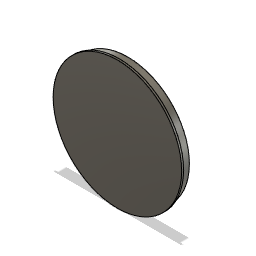
Big_Gear_ (Autodesk Fusion 360 design; units mm, degrees)
description: Spur Gear; Module: 3.0; Num Teeth: 45; Pressure Angle: 20.0; Backlash: 0.00 mm
Autodesk Fusion 360 part; units mm, degrees
(part 1 of 12)
sketch "Sketch1" plane through (0, 0, 0) normal (0, 0, 1) x (1, 0, 0) in component "Spur Gear (45 teeth)"
  circle A0 centre (0, 0) radius 63.8492
  circle A1 centre (0, 0) radius 25
extrude "Extrude1" add sketch "Sketch1" along normal blind 13 makes body 1 in component "Spur Gear (45 teeth)"
sketch "Sketch2" plane through (0, 0, 0) normal (0, 0, 1) x (1, 0, 0) in component "Spur Gear (45 teeth)"
  spline S0 degree 5 poles (63.3506, -3.1582) (63.3712, -3.1583) (63.4125, -3.1583) (63.4745, -3.1579) (63.5571, -3.1563) (63.6604, -3.1526) (63.7637, -3.1473) (63.867, -3.1403) (63.9704, -3.1319) (64.0737, -3.1219) (64.177, -3.1108) (64.2803, -3.0985) (64.3836, -3.0852) (64.4868, -3.071) (64.5901, -3.056) (64.6933, -3.0402) (64.7964, -3.0235) (64.8996, -3.0061) (65.0027, -2.9878) (65.1058, -2.9688) (65.2088, -2.949) (65.3118, -2.9284) (65.4148, -2.9072) (65.5177, -2.8853) (65.6206, -2.8627) (65.7234, -2.8395) (65.8262, -2.8156) (65.9289, -2.7911) (66.0316, -2.766) (66.1343, -2.7402) (66.2369, -2.7139) (66.3394, -2.687) (66.4419, -2.6594) (66.5443, -2.6314) (66.6467, -2.6027) (66.7491, -2.5735) (66.8514, -2.5438) (66.9536, -2.5135) (67.0558, -2.4827) (67.1579, -2.4514) (67.2599, -2.4195) (67.3619, -2.3871) (67.4639, -2.3542) (67.5657, -2.3208) (67.6675, -2.287) (67.7693, -2.2526) (67.871, -2.2177) (67.9726, -2.1824) (68.0742, -2.1465) (68.1757, -2.1102) (68.2771, -2.0735) (68.3785, -2.0362) (68.4798, -1.9985) (68.581, -1.9604) (68.6822, -1.9218) (68.7833, -1.8827) (68.8843, -1.8432) (68.9852, -1.8033) (69.0861, -1.7629) (69.1869, -1.7221) (69.2876, -1.6808) (69.3883, -1.6392) (69.4889, -1.5971) (69.5894, -1.5545) (69.6899, -1.5116) (69.7902, -1.4682) (69.8905, -1.4244) (69.9907, -1.3803) (70.0908, -1.3357) (70.1909, -1.2907) (70.2909, -1.2453) (70.3708, -1.2086) (70.4307, -1.1809) (70.4706, -1.1624) (70.4906, -1.1531) knots 0 0 0 0 0 0 0.01428571 0.02857143 0.04285714 0.05714286 0.07142857 0.08571429 0.1 0.11428571 0.12857143 0.14285714 0.15714286 0.17142857 0.18571429 0.2 0.21428571 0.22857143 0.24285714 0.25714286 0.27142857 0.28571429 0.3 0.31428571 0.32857143 0.34285714 0.35714286 0.37142857 0.38571429 0.4 0.41428571 0.42857143 0.44285714 0.45714286 0.47142857 0.48571429 0.5 0.51428571 0.52857143 0.54285714 0.55714286 0.57142857 0.58571429 0.6 0.61428571 0.62857143 0.64285714 0.65714286 0.67142857 0.68571429 0.7 0.71428571 0.72857143 0.74285714 0.75714286 0.77142857 0.78571429 0.8 0.81428571 0.82857143 0.84285714 0.85714286 0.87142857 0.88571429 0.9 0.91428571 0.92857143 0.94285714 0.95714286 0.97142857 0.98571429 1 1 1 1 1 1
  spline S1 degree 5 poles (63.3506, 3.1582) (63.3712, 3.1583) (63.4125, 3.1583) (63.4745, 3.1579) (63.5571, 3.1563) (63.6604, 3.1526) (63.7637, 3.1473) (63.867, 3.1403) (63.9704, 3.1319) (64.0737, 3.1219) (64.177, 3.1108) (64.2803, 3.0985) (64.3836, 3.0852) (64.4868, 3.071) (64.5901, 3.056) (64.6933, 3.0402) (64.7964, 3.0235) (64.8996, 3.0061) (65.0027, 2.9878) (65.1058, 2.9688) (65.2088, 2.949) (65.3118, 2.9284) (65.4148, 2.9072) (65.5177, 2.8853) (65.6206, 2.8627) (65.7234, 2.8395) (65.8262, 2.8156) (65.9289, 2.7911) (66.0316, 2.766) (66.1343, 2.7402) (66.2369, 2.7139) (66.3394, 2.687) (66.4419, 2.6594) (66.5443, 2.6314) (66.6467, 2.6027) (66.7491, 2.5735) (66.8514, 2.5438) (66.9536, 2.5135) (67.0558, 2.4827) (67.1579, 2.4514) (67.2599, 2.4195) (67.3619, 2.3871) (67.4639, 2.3542) (67.5657, 2.3208) (67.6675, 2.287) (67.7693, 2.2526) (67.871, 2.2177) (67.9726, 2.1824) (68.0742, 2.1465) (68.1757, 2.1102) (68.2771, 2.0735) (68.3785, 2.0362) (68.4798, 1.9985) (68.581, 1.9604) (68.6822, 1.9218) (68.7833, 1.8827) (68.8843, 1.8432) (68.9852, 1.8033) (69.0861, 1.7629) (69.1869, 1.7221) (69.2876, 1.6808) (69.3883, 1.6392) (69.4889, 1.5971) (69.5894, 1.5545) (69.6899, 1.5116) (69.7902, 1.4682) (69.8905, 1.4244) (69.9907, 1.3803) (70.0908, 1.3357) (70.1909, 1.2907) (70.2909, 1.2453) (70.3708, 1.2086) (70.4307, 1.1809) (70.4706, 1.1624) (70.4906, 1.1531) knots 0 0 0 0 0 0 0.01428571 0.02857143 0.04285714 0.05714286 0.07142857 0.08571429 0.1 0.11428571 0.12857143 0.14285714 0.15714286 0.17142857 0.18571429 0.2 0.21428571 0.22857143 0.24285714 0.25714286 0.27142857 0.28571429 0.3 0.31428571 0.32857143 0.34285714 0.35714286 0.37142857 0.38571429 0.4 0.41428571 0.42857143 0.44285714 0.45714286 0.47142857 0.48571429 0.5 0.51428571 0.52857143 0.54285714 0.55714286 0.57142857 0.58571429 0.6 0.61428571 0.62857143 0.64285714 0.65714286 0.67142857 0.68571429 0.7 0.71428571 0.72857143 0.74285714 0.75714286 0.77142857 0.78571429 0.8 0.81428571 0.82857143 0.84285714 0.85714286 0.87142857 0.88571429 0.9 0.91428571 0.92857143 0.94285714 0.95714286 0.97142857 0.98571429 1 1 1 1 1 1
  arc A0 (70.4906, -1.1531) -> (70.4906, 1.1531) centre (0, 0) ccw
  line L0 (63.3506, 3.1582) -> (63.3506, -3.1582)
  point P0 (63.8571, -3.1407)
  point P1 (64.3654, -3.0874)
  point P2 (64.8746, -3.0102)
  point P3 (65.3846, -2.9133)
  point P4 (65.8951, -2.7991)
  point P5 (66.406, -2.669)
  point P6 (66.917, -2.5243)
  point P7 (67.4282, -2.3657)
  point P8 (67.9393, -2.1939)
  point P9 (68.4503, -2.0094)
  point P10 (68.961, -1.8128)
  point P11 (69.4714, -1.6043)
  point P12 (69.9813, -1.3843)
  point P13 (63.8571, 3.1407)
  point P14 (64.3654, 3.0874)
  point P15 (64.8746, 3.0102)
  point P16 (65.3846, 2.9133)
  point P17 (65.8951, 2.7991)
  point P18 (66.406, 2.669)
  point P19 (66.917, 2.5243)
  point P20 (67.4282, 2.3657)
  point P21 (67.9393, 2.1939)
  point P22 (68.4503, 2.0094)
  point P23 (68.961, 1.8128)
  point P24 (69.4714, 1.6043)
  point P25 (69.9813, 1.3843)
extrude "Extrude2" add sketch "Sketch2" along normal blind 13 bodies 1 in component "Spur Gear (45 teeth)"
fillet "Fillet1" radius 1.5 2 edges at (63.7716, 3.1464, 6.5) (63.7716, -3.1464, 6.5) on bodies 1 in component "Spur Gear (45 teeth)"
pattern_circular "C-Pattern1" count 45 over 360 about axis through (0, 0, -0.0007) along (0, 0, 1) of "Extrude2", "Fillet1" in component "Spur Gear (45 teeth)"
sketch "Sketch3" plane through (0, 0, 0) normal (0, 0, 1) x (1, 0, 0) in component "Spur Gear (45 teeth)"
  circle A0 centre (0, 0) radius 67.5 construction
sketch "Sketch1 (2)" plane through (0, 0, 13) normal (0, 0, 1) x (1, 0, 0)
  arc A0 (63.688, -4.5336) -> (63.6992, -4.3741) centre (0, 0) ccw
  spline S0 degree 3 poles (64.9358, -2.9996) (64.7435, -3.0334) (64.5596, -3.1045) (64.2293, -3.3132) (64.0861, -3.4487) (63.8933, -3.7201) (63.8294, -3.8426) (63.7369, -4.1016) (63.7086, -4.2369) (63.6992, -4.3741) knots 0 0 0 0 0.058597 0.058597 0.117193 0.117193 0.158456 0.158456 0.199718 0.199718 0.199718 0.199718
  spline S1 degree 5 poles (64.9358, -2.9996) (64.9492, -2.9972) (64.9832, -2.9912) (65.0378, -2.9814) (65.113, -2.9674) (65.2088, -2.949) (65.3118, -2.9284) (65.4148, -2.9072) (65.5177, -2.8853) (65.6206, -2.8627) (65.7234, -2.8395) (65.8262, -2.8156) (65.9289, -2.7911) (66.0316, -2.766) (66.1343, -2.7402) (66.2369, -2.7139) (66.3394, -2.687) (66.4419, -2.6594) (66.5443, -2.6314) (66.6467, -2.6027) (66.7491, -2.5735) (66.8514, -2.5438) (66.9536, -2.5135) (67.0558, -2.4827) (67.1579, -2.4514) (67.2599, -2.4195) (67.3619, -2.3871) (67.4639, -2.3542) (67.5657, -2.3208) (67.6675, -2.287) (67.7693, -2.2526) (67.871, -2.2177) (67.9726, -2.1824) (68.0742, -2.1465) (68.1757, -2.1102) (68.2771, -2.0735) (68.3785, -2.0362) (68.4798, -1.9985) (68.581, -1.9604) (68.6822, -1.9218) (68.7833, -1.8827) (68.8843, -1.8432) (68.9852, -1.8033) (69.0861, -1.7629) (69.1869, -1.7221) (69.2876, -1.6808) (69.3883, -1.6392) (69.4889, -1.5971) (69.5894, -1.5545) (69.6899, -1.5116) (69.7902, -1.4682) (69.8905, -1.4244) (69.9907, -1.3803) (70.0908, -1.3357) (70.1909, -1.2907) (70.2909, -1.2453) (70.3708, -1.2086) (70.4307, -1.1809) (70.4706, -1.1624) (70.4906, -1.1531) knots 0.21931 0.21931 0.21931 0.21931 0.21931 0.21931 0.228571 0.242857 0.257143 0.271429 0.285714 0.3 0.314286 0.328571 0.342857 0.357143 0.371429 0.385714 0.4 0.414286 0.428571 0.442857 0.457143 0.471429 0.485714 0.5 0.514286 0.528571 0.542857 0.557143 0.571429 0.585714 0.6 0.614286 0.628571 0.642857 0.657143 0.671429 0.685714 0.7 0.714286 0.728571 0.742857 0.757143 0.771429 0.785714 0.8 0.814286 0.828571 0.842857 0.857143 0.871429 0.885714 0.9 0.914286 0.928571 0.942857 0.957143 0.971429 0.985714 1 1 1 1 1 1
  arc A1 (70.4906, -1.1531) -> (70.4906, 1.1531) centre (0, 0) ccw
  spline S2 degree 5 poles (70.4906, 1.1531) (70.4706, 1.1624) (70.4307, 1.1809) (70.3708, 1.2086) (70.2909, 1.2453) (70.1909, 1.2907) (70.0908, 1.3357) (69.9907, 1.3803) (69.8905, 1.4244) (69.7902, 1.4682) (69.6899, 1.5116) (69.5894, 1.5545) (69.4889, 1.5971) (69.3883, 1.6392) (69.2876, 1.6808) (69.1869, 1.7221) (69.0861, 1.7629) (68.9852, 1.8033) (68.8843, 1.8432) (68.7833, 1.8827) (68.6822, 1.9218) (68.581, 1.9604) (68.4798, 1.9985) (68.3785, 2.0362) (68.2771, 2.0735) (68.1757, 2.1102) (68.0742, 2.1465) (67.9726, 2.1824) (67.871, 2.2177) (67.7693, 2.2526) (67.6675, 2.287) (67.5657, 2.3208) (67.4639, 2.3542) (67.3619, 2.3871) (67.2599, 2.4195) (67.1579, 2.4514) (67.0558, 2.4827) (66.9536, 2.5135) (66.8514, 2.5438) (66.7491, 2.5735) (66.6467, 2.6027) (66.5443, 2.6314) (66.4419, 2.6594) (66.3394, 2.687) (66.2369, 2.7139) (66.1343, 2.7402) (66.0316, 2.766) (65.9289, 2.7911) (65.8262, 2.8156) (65.7234, 2.8395) (65.6206, 2.8627) (65.5177, 2.8853) (65.4148, 2.9072) (65.3118, 2.9284) (65.2088, 2.949) (65.113, 2.9674) (65.0378, 2.9814) (64.9832, 2.9912) (64.9492, 2.9972) (64.9358, 2.9996) knots -1 -1 -1 -1 -1 -1 -0.985714 -0.971429 -0.957143 -0.942857 -0.928571 -0.914286 -0.9 -0.885714 -0.871429 -0.857143 -0.842857 -0.828571 -0.814286 -0.8 -0.785714 -0.771429 -0.757143 -0.742857 -0.728571 -0.714286 -0.7 -0.685714 -0.671429 -0.657143 -0.642857 -0.628571 -0.614286 -0.6 -0.585714 -0.571429 -0.557143 -0.542857 -0.528571 -0.514286 -0.5 -0.485714 -0.471429 -0.457143 -0.442857 -0.428571 -0.414286 -0.4 -0.385714 -0.371429 -0.357143 -0.342857 -0.328571 -0.314286 -0.3 -0.285714 -0.271429 -0.257143 -0.242857 -0.228571 -0.21931 -0.21931 -0.21931 -0.21931 -0.21931 -0.21931
  spline S3 degree 3 poles (63.6992, 4.3741) (63.7126, 4.1793) (63.7639, 3.9889) (63.9366, 3.6385) (64.0564, 3.4818) (64.3059, 3.2615) (64.421, 3.1851) (64.6688, 3.0657) (64.8004, 3.0234) (64.9358, 2.9996) knots 0 0 0 0 0.058597 0.058597 0.117193 0.117193 0.158456 0.158456 0.199718 0.199718 0.199718 0.199718
  arc A2 (63.6992, 4.3741) -> (63.688, 4.5336) centre (0, 0) ccw
  spline S4 degree 3 poles (64.7214, 6.0669) (64.5356, 6.0067) (64.3633, 5.9107) (64.0653, 5.6581) (63.9424, 5.5039) (63.7892, 5.2084) (63.743, 5.0781) (63.6874, 4.8087) (63.6783, 4.6708) (63.688, 4.5336) knots 0 0 0 0 0.058597 0.058597 0.117193 0.117193 0.158456 0.158456 0.199718 0.199718 0.199718 0.199718
  spline S5 degree 5 poles (64.7214, 6.0669) (64.7343, 6.0711) (64.7671, 6.0818) (64.8198, 6.0992) (64.8923, 6.1235) (64.9846, 6.155) (65.0838, 6.1897) (65.1828, 6.2251) (65.2816, 6.2611) (65.3804, 6.2978) (65.4789, 6.3351) (65.5774, 6.373) (65.6757, 6.4116) (65.7739, 6.4508) (65.872, 6.4905) (65.9699, 6.5309) (66.0677, 6.5718) (66.1654, 6.6134) (66.263, 6.6554) (66.3604, 6.698) (66.4576, 6.7412) (66.5548, 6.7849) (66.6518, 6.8291) (66.7487, 6.8738) (66.8455, 6.9191) (66.9421, 6.9648) (67.0386, 7.0111) (67.1349, 7.0578) (67.2312, 7.1051) (67.3273, 7.1528) (67.4233, 7.201) (67.5191, 7.2497) (67.6148, 7.2988) (67.7104, 7.3485) (67.8059, 7.3985) (67.9012, 7.4491) (67.9964, 7.5) (68.0915, 7.5515) (68.1864, 7.6033) (68.2812, 7.6556) (68.3759, 7.7084) (68.4704, 7.7616) (68.5648, 7.8152) (68.6591, 7.8692) (68.7533, 7.9236) (68.8473, 7.9785) (68.9412, 8.0338) (69.0349, 8.0895) (69.1285, 8.1456) (69.222, 8.2021) (69.3154, 8.259) (69.4086, 8.3163) (69.5017, 8.374) (69.5946, 8.4321) (69.6874, 8.4906) (69.7801, 8.5495) (69.8542, 8.5969) (69.9096, 8.6326) (69.9466, 8.6565) (69.965, 8.6685) knots 0.21931 0.21931 0.21931 0.21931 0.21931 0.21931 0.228571 0.242857 0.257143 0.271429 0.285714 0.3 0.314286 0.328571 0.342857 0.357143 0.371429 0.385714 0.4 0.414286 0.428571 0.442857 0.457143 0.471429 0.485714 0.5 0.514286 0.528571 0.542857 0.557143 0.571429 0.585714 0.6 0.614286 0.628571 0.642857 0.657143 0.671429 0.685714 0.7 0.714286 0.728571 0.742857 0.757143 0.771429 0.785714 0.8 0.814286 0.828571 0.842857 0.857143 0.871429 0.885714 0.9 0.914286 0.928571 0.942857 0.957143 0.971429 0.985714 1 1 1 1 1 1
  arc A3 (69.965, 8.6685) -> (69.6441, 10.9523) centre (0, 0) ccw
  spline S6 degree 5 poles (69.6441, 10.9523) (69.623, 10.9587) (69.5809, 10.9715) (69.5177, 10.9906) (69.4335, 11.0157) (69.3282, 11.0468) (69.2228, 11.0774) (69.1175, 11.1076) (69.0121, 11.1375) (68.9067, 11.1669) (68.8013, 11.1958) (68.6958, 11.2244) (68.5904, 11.2525) (68.4849, 11.2802) (68.3794, 11.3075) (68.2739, 11.3343) (68.1684, 11.3607) (68.0629, 11.3866) (67.9574, 11.4121) (67.8518, 11.4372) (67.7463, 11.4618) (67.6407, 11.4859) (67.5352, 11.5096) (67.4296, 11.5329) (67.3241, 11.5556) (67.2185, 11.5779) (67.1129, 11.5997) (67.0074, 11.6211) (66.9018, 11.6419) (66.7963, 11.6623) (66.6907, 11.6822) (66.5852, 11.7016) (66.4797, 11.7205) (66.3741, 11.7389) (66.2686, 11.7567) (66.1631, 11.7741) (66.0576, 11.7909) (65.9522, 11.8072) (65.8467, 11.8229) (65.7413, 11.8382) (65.6359, 11.8528) (65.5305, 11.8669) (65.4252, 11.8805) (65.3198, 11.8935) (65.2145, 11.9059) (65.1093, 11.9177) (65.004, 11.9289) (64.8989, 11.9395) (64.7937, 11.9494) (64.6886, 11.9588) (64.5835, 11.9674) (64.4785, 11.9755) (64.3735, 11.9829) (64.2686, 11.9896) (64.1638, 11.9956) (64.0664, 12.0005) (63.9899, 12.0039) (63.9345, 12.006) (63.9, 12.0072) (63.8864, 12.0077) knots -1 -1 -1 -1 -1 -1 -0.985714 -0.971429 -0.957143 -0.942857 -0.928571 -0.914286 -0.9 -0.885714 -0.871429 -0.857143 -0.842857 -0.828571 -0.814286 -0.8 -0.785714 -0.771429 -0.757143 -0.742857 -0.728571 -0.714286 -0.7 -0.685714 -0.671429 -0.657143 -0.642857 -0.628571 -0.614286 -0.6 -0.585714 -0.571429 -0.557143 -0.542857 -0.528571 -0.514286 -0.5 -0.485714 -0.471429 -0.457143 -0.442857 -0.428571 -0.414286 -0.4 -0.385714 -0.371429 -0.357143 -0.342857 -0.328571 -0.314286 -0.3 -0.285714 -0.271429 -0.257143 -0.242857 -0.228571 -0.21931 -0.21931 -0.21931 -0.21931 -0.21931 -0.21931
  spline S7 degree 3 poles (62.4705, 13.1968) (62.5109, 13.0057) (62.5882, 12.8243) (62.808, 12.5013) (62.9484, 12.3629) (63.2261, 12.1794) (63.3508, 12.1198) (63.6128, 12.0361) (63.749, 12.0124) (63.8864, 12.0077) knots 0 0 0 0 0.058597 0.058597 0.117193 0.117193 0.158456 0.158456 0.199718 0.199718 0.199718 0.199718
  arc A4 (62.4705, 13.1968) -> (62.4373, 13.3532) centre (0, 0) ccw
  spline S8 degree 3 poles (63.2471, 15.0154) (63.0715, 14.9298) (62.9143, 14.8108) (62.6544, 14.5192) (62.5542, 14.3494) (62.4436, 14.0354) (62.416, 13.9) (62.3984, 13.6255) (62.4085, 13.4877) (62.4373, 13.3532) knots 0 0 0 0 0.058597 0.058597 0.117193 0.117193 0.158456 0.158456 0.199718 0.199718 0.199718 0.199718
  spline S9 degree 5 poles (63.2471, 15.0154) (63.2593, 15.0213) (63.2904, 15.0365) (63.3401, 15.061) (63.4086, 15.0951) (63.4956, 15.1392) (63.5889, 15.1874) (63.682, 15.2362) (63.7749, 15.2856) (63.8676, 15.3357) (63.96, 15.3864) (64.0523, 15.4376) (64.1443, 15.4895) (64.2361, 15.542) (64.3276, 15.595) (64.419, 15.6486) (64.5102, 15.7027) (64.6011, 15.7574) (64.6918, 15.8127) (64.7824, 15.8684) (64.8727, 15.9247) (64.9628, 15.9815) (65.0527, 16.0388) (65.1425, 16.0965) (65.232, 16.1548) (65.3213, 16.2136) (65.4104, 16.2728) (65.4993, 16.3325) (65.5881, 16.3927) (65.6766, 16.4533) (65.7649, 16.5144) (65.8531, 16.576) (65.941, 16.638) (66.0288, 16.7004) (66.1163, 16.7633) (66.2037, 16.8266) (66.2909, 16.8903) (66.3779, 16.9545) (66.4646, 17.019) (66.5512, 17.084) (66.6377, 17.1494) (66.7239, 17.2153) (66.8099, 17.2815) (66.8957, 17.3481) (66.9814, 17.4151) (67.0669, 17.4825) (67.1521, 17.5503) (67.2372, 17.6185) (67.3221, 17.6871) (67.4068, 17.7561) (67.4914, 17.8254) (67.5757, 17.8952) (67.6598, 17.9653) (67.7438, 18.0357) (67.8276, 18.1066) (67.9112, 18.1778) (67.9779, 18.235) (68.0278, 18.2781) (68.0611, 18.307) (68.0777, 18.3214) knots 0.21931 0.21931 0.21931 0.21931 0.21931 0.21931 0.228571 0.242857 0.257143 0.271429 0.285714 0.3 0.314286 0.328571 0.342857 0.357143 0.371429 0.385714 0.4 0.414286 0.428571 0.442857 0.457143 0.471429 0.485714 0.5 0.514286 0.528571 0.542857 0.557143 0.571429 0.585714 0.6 0.614286 0.628571 0.642857 0.657143 0.671429 0.685714 0.7 0.714286 0.728571 0.742857 0.757143 0.771429 0.785714 0.8 0.814286 0.828571 0.842857 0.857143 0.871429 0.885714 0.9 0.914286 0.928571 0.942857 0.957143 0.971429 0.985714 1 1 1 1 1 1
  arc A5 (68.0777, 18.3214) -> (67.442, 20.5383) centre (0, 0) ccw
  spline S10 degree 5 poles (67.442, 20.5383) (67.4203, 20.5417) (67.3768, 20.5485) (67.3116, 20.5586) (67.2247, 20.5718) (67.1161, 20.5879) (67.0075, 20.6036) (66.8989, 20.6188) (66.7904, 20.6337) (66.682, 20.6481) (66.5735, 20.6622) (66.4652, 20.6758) (66.3568, 20.6889) (66.2485, 20.7017) (66.1403, 20.714) (66.0321, 20.7259) (65.9239, 20.7373) (65.8158, 20.7483) (65.7078, 20.7589) (65.5998, 20.769) (65.4918, 20.7787) (65.3839, 20.7879) (65.2761, 20.7967) (65.1683, 20.805) (65.0606, 20.8129) (64.953, 20.8202) (64.8454, 20.8272) (64.7379, 20.8336) (64.6305, 20.8396) (64.5231, 20.8451) (64.4159, 20.8501) (64.3086, 20.8546) (64.2015, 20.8586) (64.0945, 20.8621) (63.9875, 20.8651) (63.8806, 20.8676) (63.7738, 20.8696) (63.6671, 20.8711) (63.5605, 20.872) (63.454, 20.8724) (63.3475, 20.8722) (63.2412, 20.8715) (63.135, 20.8703) (63.0289, 20.8685) (62.9229, 20.8661) (62.817, 20.8632) (62.7113, 20.8596) (62.6056, 20.8554) (62.5001, 20.8507) (62.3947, 20.8453) (62.2895, 20.8393) (62.1844, 20.8326) (62.0794, 20.8253) (61.9745, 20.8174) (61.8699, 20.8087) (61.7727, 20.8) (61.6966, 20.7927) (61.6414, 20.7871) (61.607, 20.7835) (61.5935, 20.7821) knots -1 -1 -1 -1 -1 -1 -0.985714 -0.971429 -0.957143 -0.942857 -0.928571 -0.914286 -0.9 -0.885714 -0.871429 -0.857143 -0.842857 -0.828571 -0.814286 -0.8 -0.785714 -0.771429 -0.757143 -0.742857 -0.728571 -0.714286 -0.7 -0.685714 -0.671429 -0.657143 -0.642857 -0.628571 -0.614286 -0.6 -0.585714 -0.571429 -0.557143 -0.542857 -0.528571 -0.514286 -0.5 -0.485714 -0.471429 -0.457143 -0.442857 -0.428571 -0.414286 -0.4 -0.385714 -0.371429 -0.357143 -0.342857 -0.328571 -0.314286 -0.3 -0.285714 -0.271429 -0.257143 -0.242857 -0.228571 -0.21931 -0.21931 -0.21931 -0.21931 -0.21931 -0.21931
  spline S11 degree 3 poles (60.0259, 21.7626) (60.0925, 21.5789) (60.1943, 21.4101) (60.4569, 21.1209) (60.6152, 21.0033) (60.9158, 20.8603) (61.0475, 20.8185) (61.3186, 20.7721) (61.4568, 20.7677) (61.5935, 20.7821) knots 0 0 0 0 0.058597 0.058597 0.117193 0.117193 0.158456 0.158456 0.199718 0.199718 0.199718 0.199718
  arc A6 (60.0259, 21.7626) -> (59.9712, 21.9128) centre (0, 0) ccw
  spline S12 degree 3 poles (60.5419, 23.6715) (60.3799, 23.5624) (60.2408, 23.4226) (60.024, 23.0977) (59.9483, 22.9156) (59.8825, 22.5893) (59.874, 22.4514) (59.8948, 22.1771) (59.924, 22.042) (59.9712, 21.9128) knots 0 0 0 0 0.058597 0.058597 0.117193 0.117193 0.158456 0.158456 0.199718 0.199718 0.199718 0.199718
  spline S13 degree 5 poles (60.5419, 23.6715) (60.5531, 23.6791) (60.5817, 23.6985) (60.6276, 23.7297) (60.6907, 23.773) (60.7707, 23.8288) (60.8564, 23.8894) (60.9418, 23.9507) (61.0269, 24.0126) (61.1117, 24.0751) (61.1962, 24.1381) (61.2804, 24.2017) (61.3643, 24.2659) (61.4479, 24.3306) (61.5312, 24.3959) (61.6142, 24.4617) (61.6969, 24.528) (61.7794, 24.5948) (61.8616, 24.6621) (61.9434, 24.73) (62.0251, 24.7983) (62.1064, 24.867) (62.1875, 24.9363) (62.2683, 25.006) (62.3488, 25.0761) (62.4291, 25.1468) (62.5091, 25.2178) (62.5889, 25.2893) (62.6683, 25.3613) (62.7476, 25.4336) (62.8265, 25.5064) (62.9053, 25.5796) (62.9837, 25.6533) (63.0619, 25.7273) (63.1399, 25.8018) (63.2176, 25.8766) (63.2951, 25.9518) (63.3723, 26.0275) (63.4492, 26.1035) (63.5259, 26.1799) (63.6024, 26.2567) (63.6786, 26.3339) (63.7546, 26.4114) (63.8303, 26.4894) (63.9058, 26.5677) (63.9811, 26.6463) (64.0561, 26.7253) (64.1309, 26.8047) (64.2054, 26.8844) (64.2797, 26.9645) (64.3537, 27.045) (64.4275, 27.1257) (64.5011, 27.2069) (64.5744, 27.2883) (64.6475, 27.3701) (64.7204, 27.4523) (64.7785, 27.5183) (64.822, 27.5679) (64.8509, 27.6011) (64.8654, 27.6177) knots 0.21931 0.21931 0.21931 0.21931 0.21931 0.21931 0.228571 0.242857 0.257143 0.271429 0.285714 0.3 0.314286 0.328571 0.342857 0.357143 0.371429 0.385714 0.4 0.414286 0.428571 0.442857 0.457143 0.471429 0.485714 0.5 0.514286 0.528571 0.542857 0.557143 0.571429 0.585714 0.6 0.614286 0.628571 0.642857 0.657143 0.671429 0.685714 0.7 0.714286 0.728571 0.742857 0.757143 0.771429 0.785714 0.8 0.814286 0.828571 0.842857 0.857143 0.871429 0.885714 0.9 0.914286 0.928571 0.942857 0.957143 0.971429 0.985714 1 1 1 1 1 1
  arc A7 (64.8654, 27.6177) -> (63.9273, 29.7245) centre (0, 0) ccw
  spline S14 degree 5 poles (63.9273, 29.7245) (63.9053, 29.7249) (63.8613, 29.7256) (63.7953, 29.7265) (63.7074, 29.7275) (63.5976, 29.7283) (63.4879, 29.7287) (63.3783, 29.7287) (63.2688, 29.7283) (63.1594, 29.7275) (63.05, 29.7263) (62.9408, 29.7247) (62.8317, 29.7227) (62.7227, 29.7202) (62.6138, 29.7173) (62.505, 29.7141) (62.3963, 29.7103) (62.2877, 29.7062) (62.1792, 29.7016) (62.0709, 29.6966) (61.9626, 29.6912) (61.8545, 29.6853) (61.7465, 29.679) (61.6386, 29.6722) (61.5309, 29.665) (61.4233, 29.6573) (61.3158, 29.6492) (61.2084, 29.6406) (61.1012, 29.6316) (60.9941, 29.6221) (60.8872, 29.6121) (60.7804, 29.6017) (60.6737, 29.5907) (60.5672, 29.5793) (60.4609, 29.5674) (60.3547, 29.555) (60.2487, 29.5421) (60.1428, 29.5287) (60.0371, 29.5148) (59.9316, 29.5003) (59.8262, 29.4854) (59.721, 29.4699) (59.616, 29.4539) (59.5112, 29.4373) (59.4065, 29.4202) (59.3021, 29.4026) (59.1979, 29.3843) (59.0938, 29.3655) (58.99, 29.3461) (58.8864, 29.3261) (58.783, 29.3055) (58.6798, 29.2843) (58.5769, 29.2624) (58.4742, 29.24) (58.3717, 29.2168) (58.2767, 29.1947) (58.2024, 29.1769) (58.1485, 29.1636) (58.115, 29.1553) (58.1018, 29.152) knots -1 -1 -1 -1 -1 -1 -0.985714 -0.971429 -0.957143 -0.942857 -0.928571 -0.914286 -0.9 -0.885714 -0.871429 -0.857143 -0.842857 -0.828571 -0.814286 -0.8 -0.785714 -0.771429 -0.757143 -0.742857 -0.728571 -0.714286 -0.7 -0.685714 -0.671429 -0.657143 -0.642857 -0.628571 -0.614286 -0.6 -0.585714 -0.571429 -0.557143 -0.542857 -0.528571 -0.514286 -0.5 -0.485714 -0.471429 -0.457143 -0.442857 -0.428571 -0.414286 -0.4 -0.385714 -0.371429 -0.357143 -0.342857 -0.328571 -0.314286 -0.3 -0.285714 -0.271429 -0.257143 -0.242857 -0.228571 -0.21931 -0.21931 -0.21931 -0.21931 -0.21931 -0.21931
  spline S15 degree 3 poles (56.413, 29.9048) (56.5045, 29.7322) (56.6288, 29.5791) (56.9291, 29.3293) (57.1022, 29.2349) (57.4198, 29.1351) (57.556, 29.1121) (57.831, 29.1039) (57.9684, 29.1187) (58.1018, 29.152) knots 0 0 0 0 0.058597 0.058597 0.117193 0.117193 0.158456 0.158456 0.199718 0.199718 0.199718 0.199718
  arc A8 (56.413, 29.9048) -> (56.3379, 30.046) centre (0, 0) ccw
  spline S16 degree 3 poles (56.6583, 31.867) (56.513, 31.7363) (56.3947, 31.5786) (56.2252, 31.2266) (56.1757, 31.0358) (56.1559, 30.7035) (56.1667, 30.5657) (56.2255, 30.297) (56.2732, 30.1673) (56.3379, 30.046) knots 0 0 0 0 0.058597 0.058597 0.117193 0.117193 0.158456 0.158456 0.199718 0.199718 0.199718 0.199718
  spline S17 degree 5 poles (56.6583, 31.867) (56.6683, 31.8761) (56.694, 31.8992) (56.7351, 31.9365) (56.7915, 31.9881) (56.8629, 32.0545) (56.9394, 32.1265) (57.0154, 32.1991) (57.0911, 32.2722) (57.1664, 32.3459) (57.2413, 32.4201) (57.3158, 32.4948) (57.3899, 32.57) (57.4637, 32.6457) (57.5371, 32.722) (57.6102, 32.7987) (57.6829, 32.8759) (57.7552, 32.9535) (57.8272, 33.0316) (57.8989, 33.1102) (57.9702, 33.1891) (58.0412, 33.2686) (58.1118, 33.3484) (58.1821, 33.4287) (58.2521, 33.5094) (58.3218, 33.5905) (58.3911, 33.672) (58.4601, 33.7539) (58.5288, 33.8362) (58.5972, 33.9189) (58.6653, 34.002) (58.7331, 34.0854) (58.8005, 34.1693) (58.8677, 34.2535) (58.9345, 34.338) (59.001, 34.423) (59.0673, 34.5082) (59.1332, 34.5939) (59.1988, 34.6799) (59.2642, 34.7662) (59.3292, 34.8529) (59.3939, 34.94) (59.4584, 35.0273) (59.5225, 35.115) (59.5864, 35.2031) (59.65, 35.2914) (59.7132, 35.3801) (59.7762, 35.4691) (59.8389, 35.5585) (59.9014, 35.6481) (59.9635, 35.7381) (60.0253, 35.8283) (60.0869, 35.9189) (60.1482, 36.0098) (60.2092, 36.101) (60.2699, 36.1925) (60.3183, 36.2659) (60.3544, 36.3211) (60.3785, 36.358) (60.3905, 36.3764) knots 0.21931 0.21931 0.21931 0.21931 0.21931 0.21931 0.228571 0.242857 0.257143 0.271429 0.285714 0.3 0.314286 0.328571 0.342857 0.357143 0.371429 0.385714 0.4 0.414286 0.428571 0.442857 0.457143 0.471429 0.485714 0.5 0.514286 0.528571 0.542857 0.557143 0.571429 0.585714 0.6 0.614286 0.628571 0.642857 0.657143 0.671429 0.685714 0.7 0.714286 0.728571 0.742857 0.757143 0.771429 0.785714 0.8 0.814286 0.828571 0.842857 0.857143 0.871429 0.885714 0.9 0.914286 0.928571 0.942857 0.957143 0.971429 0.985714 1 1 1 1 1 1
  arc A9 (60.3905, 36.3764) -> (59.1683, 38.3322) centre (0, 0) ccw
  spline S18 degree 5 poles (59.1683, 38.3322) (59.1465, 38.3295) (59.1028, 38.3241) (59.0374, 38.3158) (58.9502, 38.3045) (58.8413, 38.29) (58.7326, 38.2752) (58.6241, 38.2599) (58.5157, 38.2443) (58.4074, 38.2283) (58.2993, 38.2119) (58.1914, 38.1951) (58.0836, 38.1779) (57.976, 38.1603) (57.8686, 38.1423) (57.7613, 38.1239) (57.6541, 38.1051) (57.5472, 38.0859) (57.4404, 38.0662) (57.3338, 38.0462) (57.2274, 38.0258) (57.1211, 38.0049) (57.0151, 37.9836) (56.9092, 37.9619) (56.8035, 37.9398) (56.698, 37.9172) (56.5927, 37.8942) (56.4876, 37.8707) (56.3827, 37.8469) (56.2779, 37.8225) (56.1734, 37.7978) (56.0691, 37.7726) (55.965, 37.7469) (55.8612, 37.7208) (55.7575, 37.6942) (55.6541, 37.6671) (55.5509, 37.6396) (55.4479, 37.6116) (55.3452, 37.5831) (55.2427, 37.5541) (55.1404, 37.5246) (55.0384, 37.4947) (54.9366, 37.4642) (54.8351, 37.4332) (54.7339, 37.4017) (54.6329, 37.3697) (54.5322, 37.3371) (54.4318, 37.304) (54.3317, 37.2703) (54.2319, 37.2361) (54.1324, 37.2013) (54.0332, 37.1659) (53.9343, 37.13) (53.8357, 37.0934) (53.7375, 37.0563) (53.6465, 37.0211) (53.5753, 36.9931) (53.5238, 36.9725) (53.4918, 36.9596) (53.4792, 36.9545) knots -1 -1 -1 -1 -1 -1 -0.985714 -0.971429 -0.957143 -0.942857 -0.928571 -0.914286 -0.9 -0.885714 -0.871429 -0.857143 -0.842857 -0.828571 -0.814286 -0.8 -0.785714 -0.771429 -0.757143 -0.742857 -0.728571 -0.714286 -0.7 -0.685714 -0.671429 -0.657143 -0.642857 -0.628571 -0.614286 -0.6 -0.585714 -0.571429 -0.557143 -0.542857 -0.528571 -0.514286 -0.5 -0.485714 -0.471429 -0.457143 -0.442857 -0.428571 -0.414286 -0.4 -0.385714 -0.371429 -0.357143 -0.342857 -0.328571 -0.314286 -0.3 -0.285714 -0.271429 -0.257143 -0.242857 -0.228571 -0.21931 -0.21931 -0.21931 -0.21931 -0.21931 -0.21931
  spline S19 degree 3 poles (51.702, 37.4649) (51.8166, 37.3067) (51.9611, 37.1725) (52.2932, 36.9669) (52.4778, 36.8975) (52.8061, 36.8428) (52.9443, 36.839) (53.2177, 36.8692) (53.3517, 36.903) (53.4792, 36.9545) knots 0 0 0 0 0.058597 0.058597 0.117193 0.117193 0.158456 0.158456 0.199718 0.199718 0.199718 0.199718
  arc A10 (51.702, 37.4649) -> (51.6081, 37.5943) centre (0, 0) ccw
  spline S20 degree 3 poles (51.6718, 39.4422) (51.5462, 39.2926) (51.451, 39.1199) (51.3322, 38.7478) (51.3096, 38.5519) (51.3363, 38.2201) (51.3662, 38.0852) (51.4618, 37.8272) (51.5271, 37.7054) (51.6081, 37.5943) knots 0 0 0 0 0.058597 0.058597 0.117193 0.117193 0.158456 0.158456 0.199718 0.199718 0.199718 0.199718
  spline S21 degree 5 poles (51.6718, 39.4422) (51.6806, 39.4525) (51.7027, 39.479) (51.7382, 39.5217) (51.7869, 39.5807) (51.8484, 39.6564) (51.9141, 39.7383) (51.9793, 39.8208) (52.0441, 39.9037) (52.1084, 39.9871) (52.1722, 40.071) (52.2356, 40.1554) (52.2986, 40.2402) (52.3611, 40.3254) (52.4232, 40.4111) (52.4848, 40.4973) (52.5461, 40.5838) (52.6069, 40.6708) (52.6673, 40.7581) (52.7274, 40.8459) (52.787, 40.934) (52.8462, 41.0226) (52.9051, 41.1115) (52.9635, 41.2007) (53.0216, 41.2904) (53.0793, 41.3804) (53.1366, 41.4708) (53.1936, 41.5615) (53.2502, 41.6525) (53.3064, 41.744) (53.3622, 41.8357) (53.4177, 41.9278) (53.4728, 42.0202) (53.5276, 42.1129) (53.582, 42.2059) (53.6361, 42.2993) (53.6898, 42.393) (53.7432, 42.487) (53.7962, 42.5813) (53.8489, 42.6759) (53.9012, 42.7708) (53.9532, 42.866) (54.0049, 42.9615) (54.0562, 43.0572) (54.1072, 43.1533) (54.1578, 43.2496) (54.2082, 43.3463) (54.2582, 43.4432) (54.3078, 43.5404) (54.3572, 43.6378) (54.4062, 43.7356) (54.4548, 43.8336) (54.5032, 43.9318) (54.5512, 44.0304) (54.599, 44.1291) (54.6464, 44.2282) (54.684, 44.3076) (54.7121, 44.3673) (54.7308, 44.4072) (54.7401, 44.4271) knots 0.21931 0.21931 0.21931 0.21931 0.21931 0.21931 0.228571 0.242857 0.257143 0.271429 0.285714 0.3 0.314286 0.328571 0.342857 0.357143 0.371429 0.385714 0.4 0.414286 0.428571 0.442857 0.457143 0.471429 0.485714 0.5 0.514286 0.528571 0.542857 0.557143 0.571429 0.585714 0.6 0.614286 0.628571 0.642857 0.657143 0.671429 0.685714 0.7 0.714286 0.728571 0.742857 0.757143 0.771429 0.785714 0.8 0.814286 0.828571 0.842857 0.857143 0.871429 0.885714 0.9 0.914286 0.928571 0.942857 0.957143 0.971429 0.985714 1 1 1 1 1 1
  arc A11 (54.7401, 44.4271) -> (53.2577, 46.1938) centre (0, 0) ccw
  spline S22 degree 5 poles (53.2577, 46.1938) (53.2364, 46.1881) (53.194, 46.1766) (53.1303, 46.1593) (53.0455, 46.136) (52.9397, 46.1065) (52.8342, 46.0767) (52.7288, 46.0465) (52.6236, 46.0159) (52.5187, 45.985) (52.4139, 45.9537) (52.3094, 45.9221) (52.205, 45.89) (52.1009, 45.8576) (51.997, 45.8248) (51.8933, 45.7917) (51.7899, 45.7582) (51.6866, 45.7242) (51.5836, 45.6899) (51.4808, 45.6553) (51.3783, 45.6202) (51.276, 45.5848) (51.1739, 45.5489) (51.0721, 45.5127) (50.9705, 45.476) (50.8692, 45.439) (50.7681, 45.4016) (50.6673, 45.3637) (50.5667, 45.3255) (50.4664, 45.2868) (50.3663, 45.2478) (50.2665, 45.2083) (50.167, 45.1684) (50.0678, 45.128) (49.9689, 45.0873) (49.8702, 45.0461) (49.7718, 45.0045) (49.6738, 44.9624) (49.576, 44.9199) (49.4785, 44.8769) (49.3814, 44.8335) (49.2845, 44.7896) (49.188, 44.7453) (49.0918, 44.7005) (48.9959, 44.6552) (48.9004, 44.6094) (48.8052, 44.5632) (48.7104, 44.5164) (48.6159, 44.4691) (48.5219, 44.4213) (48.4282, 44.373) (48.3348, 44.3242) (48.2419, 44.2748) (48.1494, 44.2249) (48.0573, 44.1745) (47.9721, 44.127) (47.9055, 44.0893) (47.8573, 44.0618) (47.8274, 44.0446) (47.8157, 44.0378) knots -1 -1 -1 -1 -1 -1 -0.985714 -0.971429 -0.957143 -0.942857 -0.928571 -0.914286 -0.9 -0.885714 -0.871429 -0.857143 -0.842857 -0.828571 -0.814286 -0.8 -0.785714 -0.771429 -0.757143 -0.742857 -0.728571 -0.714286 -0.7 -0.685714 -0.671429 -0.657143 -0.642857 -0.628571 -0.614286 -0.6 -0.585714 -0.571429 -0.557143 -0.542857 -0.528571 -0.514286 -0.5 -0.485714 -0.471429 -0.457143 -0.442857 -0.428571 -0.414286 -0.4 -0.385714 -0.371429 -0.357143 -0.342857 -0.328571 -0.314286 -0.3 -0.285714 -0.271429 -0.257143 -0.242857 -0.228571 -0.21931 -0.21931 -0.21931 -0.21931 -0.21931 -0.21931
  spline S23 degree 3 poles (45.9848, 44.2958) (46.1203, 44.1552) (46.282, 44.0423) (46.6395, 43.8849) (46.8319, 43.8419) (47.1647, 43.8335) (47.302, 43.8489) (47.5686, 43.9168) (47.6966, 43.9689) (47.8157, 44.0378) knots 0 0 0 0 0.058597 0.058597 0.117193 0.117193 0.158456 0.158456 0.199718 0.199718 0.199718 0.199718
  arc A12 (45.9848, 44.2958) -> (45.8737, 44.4109) centre (0, 0) ccw
  spline S24 degree 3 poles (45.6797, 46.2496) (45.5761, 46.084) (45.5059, 45.8998) (45.44, 45.5147) (45.4449, 45.3176) (45.5175, 44.9928) (45.5658, 44.8633) (45.6964, 44.6212) (45.778, 44.5097) (45.8737, 44.4109) knots 0 0 0 0 0.058597 0.058597 0.117193 0.117193 0.158456 0.158456 0.199718 0.199718 0.199718 0.199718
  spline S25 degree 5 poles (45.6797, 46.2496) (45.6869, 46.2611) (45.7051, 46.2904) (45.7344, 46.3376) (45.7743, 46.4028) (45.8247, 46.4863) (45.8784, 46.5766) (45.9315, 46.6674) (45.9841, 46.7585) (46.0361, 46.8501) (46.0877, 46.942) (46.1387, 47.0344) (46.1892, 47.1271) (46.2393, 47.2203) (46.2888, 47.3138) (46.3379, 47.4076) (46.3865, 47.5019) (46.4347, 47.5964) (46.4823, 47.6914) (46.5296, 47.7866) (46.5764, 47.8822) (46.6227, 47.9781) (46.6686, 48.0743) (46.7141, 48.1709) (46.7591, 48.2677) (46.8037, 48.3649) (46.8479, 48.4624) (46.8917, 48.5601) (46.935, 48.6582) (46.978, 48.7565) (47.0205, 48.8551) (47.0626, 48.954) (47.1044, 49.0532) (47.1457, 49.1527) (47.1866, 49.2524) (47.2272, 49.3524) (47.2673, 49.4526) (47.3071, 49.5531) (47.3465, 49.6539) (47.3855, 49.7549) (47.4241, 49.8561) (47.4624, 49.9576) (47.5002, 50.0594) (47.5377, 50.1614) (47.5748, 50.2636) (47.6116, 50.3661) (47.648, 50.4688) (47.684, 50.5717) (47.7196, 50.6748) (47.7549, 50.7782) (47.7899, 50.8818) (47.8244, 50.9856) (47.8587, 51.0897) (47.8925, 51.1939) (47.926, 51.2984) (47.9592, 51.4031) (47.9854, 51.487) (48.0049, 51.55) (48.0179, 51.5921) (48.0243, 51.6131) knots 0.21931 0.21931 0.21931 0.21931 0.21931 0.21931 0.228571 0.242857 0.257143 0.271429 0.285714 0.3 0.314286 0.328571 0.342857 0.357143 0.371429 0.385714 0.4 0.414286 0.428571 0.442857 0.457143 0.471429 0.485714 0.5 0.514286 0.528571 0.542857 0.557143 0.571429 0.585714 0.6 0.614286 0.628571 0.642857 0.657143 0.671429 0.685714 0.7 0.714286 0.728571 0.742857 0.757143 0.771429 0.785714 0.8 0.814286 0.828571 0.842857 0.857143 0.871429 0.885714 0.9 0.914286 0.928571 0.942857 0.957143 0.971429 0.985714 1 1 1 1 1 1
  arc A13 (48.0243, 51.6131) -> (46.3105, 53.1563) centre (0, 0) ccw
  spline S26 degree 5 poles (46.3105, 53.1563) (46.2902, 53.1477) (46.2497, 53.1304) (46.1891, 53.1044) (46.1084, 53.0695) (46.0077, 53.0256) (45.9073, 52.9814) (45.8072, 52.9368) (45.7073, 52.8919) (45.6077, 52.8467) (45.5083, 52.8011) (45.4092, 52.7552) (45.3103, 52.709) (45.2117, 52.6624) (45.1134, 52.6155) (45.0153, 52.5682) (44.9175, 52.5206) (44.82, 52.4726) (44.7228, 52.4243) (44.6258, 52.3757) (44.5292, 52.3267) (44.4328, 52.2774) (44.3367, 52.2277) (44.2409, 52.1776) (44.1454, 52.1272) (44.0502, 52.0764) (43.9553, 52.0253) (43.8607, 51.9738) (43.7665, 51.9219) (43.6725, 51.8697) (43.5789, 51.8171) (43.4856, 51.7641) (43.3926, 51.7107) (43.2999, 51.657) (43.2076, 51.6028) (43.1157, 51.5483) (43.0241, 51.4934) (42.9328, 51.4381) (42.8419, 51.3824) (42.7513, 51.3263) (42.6612, 51.2697) (42.5714, 51.2128) (42.482, 51.1555) (42.3929, 51.0977) (42.3043, 51.0395) (42.2161, 50.9809) (42.1283, 50.9218) (42.0409, 50.8623) (41.9539, 50.8024) (41.8674, 50.742) (41.7813, 50.6811) (41.6957, 50.6197) (41.6106, 50.5579) (41.5259, 50.4956) (41.4417, 50.4328) (41.3639, 50.374) (41.3032, 50.3274) (41.2594, 50.2934) (41.2321, 50.2722) (41.2214, 50.2638) knots -1 -1 -1 -1 -1 -1 -0.985714 -0.971429 -0.957143 -0.942857 -0.928571 -0.914286 -0.9 -0.885714 -0.871429 -0.857143 -0.842857 -0.828571 -0.814286 -0.8 -0.785714 -0.771429 -0.757143 -0.742857 -0.728571 -0.714286 -0.7 -0.685714 -0.671429 -0.657143 -0.642857 -0.628571 -0.614286 -0.6 -0.585714 -0.571429 -0.557143 -0.542857 -0.528571 -0.514286 -0.5 -0.485714 -0.471429 -0.457143 -0.442857 -0.428571 -0.414286 -0.4 -0.385714 -0.371429 -0.357143 -0.342857 -0.328571 -0.314286 -0.3 -0.285714 -0.271429 -0.257143 -0.242857 -0.228571 -0.21931 -0.21931 -0.21931 -0.21931 -0.21931 -0.21931
  spline S27 degree 3 poles (39.3725, 50.2646) (39.5262, 50.1442) (39.702, 50.0549) (40.078, 49.9488) (40.2746, 49.933) (40.6052, 49.9709) (40.7391, 50.0054) (40.9936, 50.1097) (41.1131, 50.1791) (41.2214, 50.2638) knots 0 0 0 0 0.058597 0.058597 0.117193 0.117193 0.158456 0.158456 0.199718 0.199718 0.199718 0.199718
  arc A14 (39.3725, 50.2646) -> (39.2465, 50.363) centre (0, 0) ccw
  spline S28 degree 3 poles (38.7984, 52.1569) (38.7189, 51.9785) (38.675, 51.7863) (38.6633, 51.3958) (38.6957, 51.2013) (38.8128, 50.8897) (38.8786, 50.7682) (39.0416, 50.5466) (39.138, 50.4476) (39.2465, 50.363) knots 0 0 0 0 0.058597 0.058597 0.117193 0.117193 0.158456 0.158456 0.199718 0.199718 0.199718 0.199718
  spline S29 degree 5 poles (38.7984, 52.1569) (38.8039, 52.1693) (38.818, 52.2009) (38.8403, 52.2516) (38.8708, 52.3218) (38.9091, 52.4115) (38.9497, 52.5084) (38.9896, 52.6056) (39.029, 52.7032) (39.0678, 52.8011) (39.1061, 52.8994) (39.1438, 52.9979) (39.1809, 53.0968) (39.2175, 53.196) (39.2536, 53.2955) (39.2891, 53.3953) (39.3241, 53.4953) (39.3586, 53.5957) (39.3926, 53.6963) (39.4261, 53.7972) (39.4592, 53.8984) (39.4917, 53.9998) (39.5238, 54.1015) (39.5554, 54.2034) (39.5865, 54.3056) (39.6171, 54.408) (39.6473, 54.5107) (39.6771, 54.6136) (39.7063, 54.7167) (39.7352, 54.8201) (39.7636, 54.9237) (39.7915, 55.0275) (39.8191, 55.1315) (39.8462, 55.2357) (39.8728, 55.3402) (39.8991, 55.4448) (39.9249, 55.5497) (39.9503, 55.6547) (39.9752, 55.76) (39.9998, 55.8654) (40.024, 55.9711) (40.0477, 56.0769) (40.071, 56.183) (40.094, 56.2892) (40.1165, 56.3956) (40.1386, 56.5022) (40.1604, 56.6089) (40.1817, 56.7158) (40.2027, 56.823) (40.2232, 56.9302) (40.2434, 57.0377) (40.2632, 57.1453) (40.2826, 57.2531) (40.3016, 57.3611) (40.3203, 57.4692) (40.3385, 57.5774) (40.3528, 57.6642) (40.3634, 57.7293) (40.3703, 57.7728) (40.3738, 57.7945) knots 0.21931 0.21931 0.21931 0.21931 0.21931 0.21931 0.228571 0.242857 0.257143 0.271429 0.285714 0.3 0.314286 0.328571 0.342857 0.357143 0.371429 0.385714 0.4 0.414286 0.428571 0.442857 0.457143 0.471429 0.485714 0.5 0.514286 0.528571 0.542857 0.557143 0.571429 0.585714 0.6 0.614286 0.628571 0.642857 0.657143 0.671429 0.685714 0.7 0.714286 0.728571 0.742857 0.757143 0.771429 0.785714 0.8 0.814286 0.828571 0.842857 0.857143 0.871429 0.885714 0.9 0.914286 0.928571 0.942857 0.957143 0.971429 0.985714 1 1 1 1 1 1
  arc A15 (40.3738, 57.7945) -> (38.4618, 59.0842) centre (0, 0) ccw
  spline S30 degree 5 poles (38.4618, 59.0842) (38.443, 59.0728) (38.4053, 59.0501) (38.3489, 59.0159) (38.2738, 58.9701) (38.1802, 58.9126) (38.087, 58.8548) (37.994, 58.7968) (37.9014, 58.7384) (37.809, 58.6797) (37.7169, 58.6208) (37.6251, 58.5615) (37.5337, 58.502) (37.4425, 58.4421) (37.3517, 58.382) (37.2612, 58.3215) (37.1709, 58.2608) (37.0811, 58.1997) (36.9915, 58.1384) (36.9023, 58.0767) (36.8134, 58.0147) (36.7248, 57.9525) (36.6365, 57.8899) (36.5486, 57.827) (36.4611, 57.7638) (36.3739, 57.7002) (36.287, 57.6364) (36.2005, 57.5722) (36.1144, 57.5077) (36.0286, 57.4429) (35.9432, 57.3778) (35.8582, 57.3123) (35.7736, 57.2465) (35.6893, 57.1804) (35.6054, 57.114) (35.5219, 57.0472) (35.4389, 56.98) (35.3562, 56.9126) (35.2739, 56.8448) (35.1921, 56.7766) (35.1106, 56.7081) (35.0296, 56.6392) (34.9491, 56.57) (34.8689, 56.5004) (34.7893, 56.4304) (34.7101, 56.3601) (34.6313, 56.2894) (34.5531, 56.2183) (34.4753, 56.1468) (34.398, 56.075) (34.3213, 56.0027) (34.245, 55.93) (34.1693, 55.857) (34.0941, 55.7835) (34.0195, 55.7096) (33.9506, 55.6405) (33.897, 55.5859) (33.8583, 55.5462) (33.8343, 55.5214) (33.8249, 55.5116) knots -1 -1 -1 -1 -1 -1 -0.985714 -0.971429 -0.957143 -0.942857 -0.928571 -0.914286 -0.9 -0.885714 -0.871429 -0.857143 -0.842857 -0.828571 -0.814286 -0.8 -0.785714 -0.771429 -0.757143 -0.742857 -0.728571 -0.714286 -0.7 -0.685714 -0.671429 -0.657143 -0.642857 -0.628571 -0.614286 -0.6 -0.585714 -0.571429 -0.557143 -0.542857 -0.528571 -0.514286 -0.5 -0.485714 -0.471429 -0.457143 -0.442857 -0.428571 -0.414286 -0.4 -0.385714 -0.371429 -0.357143 -0.342857 -0.328571 -0.314286 -0.3 -0.285714 -0.271429 -0.257143 -0.242857 -0.228571 -0.21931 -0.21931 -0.21931 -0.21931 -0.21931 -0.21931
  spline S31 degree 3 poles (31.9938, 55.255) (32.1628, 55.1571) (32.3494, 55.0932) (32.7364, 55.0405) (32.9333, 55.0522) (33.2555, 55.1358) (33.3832, 55.1885) (33.6207, 55.3272) (33.7294, 55.4126) (33.8249, 55.5116) knots 0 0 0 0 0.058597 0.058597 0.117193 0.117193 0.158456 0.158456 0.199718 0.199718 0.199718 0.199718
  arc A16 (31.9938, 55.255) -> (31.8553, 55.335) centre (0, 0) ccw
  spline S32 degree 3 poles (31.162, 57.049) (31.1081, 56.8613) (31.0913, 56.6648) (31.1341, 56.2765) (31.1932, 56.0884) (31.3526, 55.7962) (31.4347, 55.685) (31.6269, 55.4883) (31.7361, 55.4036) (31.8553, 55.335) knots 0 0 0 0 0.058597 0.058597 0.117193 0.117193 0.158456 0.158456 0.199718 0.199718 0.199718 0.199718
  spline S33 degree 5 poles (31.162, 57.049) (31.1657, 57.0621) (31.1752, 57.0953) (31.1903, 57.1487) (31.2108, 57.2224) (31.2362, 57.3165) (31.2629, 57.4181) (31.2889, 57.52) (31.3143, 57.6221) (31.3391, 57.7244) (31.3633, 57.8271) (31.3869, 57.9299) (31.41, 58.033) (31.4324, 58.1363) (31.4543, 58.2398) (31.4756, 58.3436) (31.4963, 58.4476) (31.5165, 58.5518) (31.5362, 58.6561) (31.5553, 58.7607) (31.5739, 58.8655) (31.5921, 58.9705) (31.6097, 59.0756) (31.6267, 59.181) (31.6433, 59.2865) (31.6594, 59.3922) (31.675, 59.498) (31.6902, 59.6041) (31.7048, 59.7103) (31.719, 59.8167) (31.7327, 59.9232) (31.7459, 60.0299) (31.7587, 60.1367) (31.771, 60.2437) (31.7829, 60.3508) (31.7943, 60.4581) (31.8053, 60.5655) (31.8158, 60.6731) (31.8259, 60.7808) (31.8356, 60.8887) (31.8448, 60.9966) (31.8536, 61.1048) (31.8619, 61.213) (31.8698, 61.3214) (31.8773, 61.4299) (31.8844, 61.5385) (31.8911, 61.6472) (31.8974, 61.7561) (31.9032, 61.8651) (31.9086, 61.9742) (31.9136, 62.0834) (31.9183, 62.1927) (31.9225, 62.3022) (31.9263, 62.4117) (31.9297, 62.5214) (31.9327, 62.6311) (31.9348, 62.719) (31.9362, 62.785) (31.9371, 62.829) (31.9375, 62.851) knots 0.21931 0.21931 0.21931 0.21931 0.21931 0.21931 0.228571 0.242857 0.257143 0.271429 0.285714 0.3 0.314286 0.328571 0.342857 0.357143 0.371429 0.385714 0.4 0.414286 0.428571 0.442857 0.457143 0.471429 0.485714 0.5 0.514286 0.528571 0.542857 0.557143 0.571429 0.585714 0.6 0.614286 0.628571 0.642857 0.657143 0.671429 0.685714 0.7 0.714286 0.728571 0.742857 0.757143 0.771429 0.785714 0.8 0.814286 0.828571 0.842857 0.857143 0.871429 0.885714 0.9 0.914286 0.928571 0.942857 0.957143 0.971429 0.985714 1 1 1 1 1 1
  arc A17 (31.9375, 62.851) -> (29.8646, 63.862) centre (0, 0) ccw
  spline S34 degree 5 poles (29.8646, 63.862) (29.8475, 63.8481) (29.8134, 63.8204) (29.7622, 63.7787) (29.6943, 63.7229) (29.6096, 63.6529) (29.5253, 63.5827) (29.4413, 63.5123) (29.3577, 63.4416) (29.2744, 63.3707) (29.1914, 63.2995) (29.1088, 63.228) (29.0265, 63.1563) (28.9446, 63.0844) (28.863, 63.0122) (28.7817, 62.9397) (28.7009, 62.867) (28.6204, 62.794) (28.5402, 62.7208) (28.4604, 62.6473) (28.381, 62.5736) (28.302, 62.4996) (28.2233, 62.4253) (28.145, 62.3508) (28.0671, 62.276) (27.9896, 62.201) (27.9125, 62.1256) (27.8357, 62.0501) (27.7594, 61.9742) (27.6835, 61.8981) (27.608, 61.8217) (27.5329, 61.7451) (27.4582, 61.6681) (27.384, 61.5909) (27.3102, 61.5135) (27.2368, 61.4357) (27.1639, 61.3577) (27.0914, 61.2793) (27.0194, 61.2007) (26.9478, 61.1218) (26.8767, 61.0427) (26.8061, 60.9632) (26.7359, 60.8834) (26.6663, 60.8033) (26.5971, 60.723) (26.5284, 60.6423) (26.4603, 60.5613) (26.3927, 60.4801) (26.3257, 60.3984) (26.2591, 60.3165) (26.1932, 60.2343) (26.1278, 60.1517) (26.063, 60.0688) (25.9987, 59.9856) (25.9351, 59.902) (25.8766, 59.824) (25.8311, 59.7625) (25.7983, 59.7178) (25.778, 59.6899) (25.77, 59.6789) knots -1 -1 -1 -1 -1 -1 -0.985714 -0.971429 -0.957143 -0.942857 -0.928571 -0.914286 -0.9 -0.885714 -0.871429 -0.857143 -0.842857 -0.828571 -0.814286 -0.8 -0.785714 -0.771429 -0.757143 -0.742857 -0.728571 -0.714286 -0.7 -0.685714 -0.671429 -0.657143 -0.642857 -0.628571 -0.614286 -0.6 -0.585714 -0.571429 -0.557143 -0.542857 -0.528571 -0.514286 -0.5 -0.485714 -0.471429 -0.457143 -0.442857 -0.428571 -0.414286 -0.4 -0.385714 -0.371429 -0.357143 -0.342857 -0.328571 -0.314286 -0.3 -0.285714 -0.271429 -0.257143 -0.242857 -0.228571 -0.21931 -0.21931 -0.21931 -0.21931 -0.21931 -0.21931
  spline S35 degree 3 poles (23.9924, 59.17) (24.1734, 59.0966) (24.3671, 59.0592) (24.7577, 59.0609) (24.951, 59.0998) (25.2584, 59.2275) (25.3776, 59.2975) (25.5935, 59.4679) (25.6892, 59.5676) (25.77, 59.6789) knots 0 0 0 0 0.058597 0.058597 0.117193 0.117193 0.158456 0.158456 0.199718 0.199718 0.199718 0.199718
  arc A18 (23.9924, 59.17) -> (23.8442, 59.2299) centre (0, 0) ccw
  spline S36 degree 3 poles (22.919, 60.8307) (22.8918, 60.6373) (22.9025, 60.4404) (22.9989, 60.0619) (23.0837, 59.8838) (23.2821, 59.6166) (23.3789, 59.518) (23.5967, 59.3499) (23.7166, 59.2812) (23.8442, 59.2299) knots 0 0 0 0 0.058597 0.058597 0.117193 0.117193 0.158456 0.158456 0.199718 0.199718 0.199718 0.199718
  spline S37 degree 5 poles (22.919, 60.8307) (22.9209, 60.8442) (22.9257, 60.8784) (22.9332, 60.9333) (22.9432, 61.0092) (22.9553, 61.106) (22.9676, 61.2103) (22.9792, 61.3148) (22.9901, 61.4194) (23.0004, 61.5242) (23.0101, 61.6292) (23.0192, 61.7343) (23.0276, 61.8396) (23.0355, 61.9451) (23.0427, 62.0506) (23.0494, 62.1564) (23.0555, 62.2622) (23.061, 62.3682) (23.0659, 62.4743) (23.0703, 62.5805) (23.0742, 62.6869) (23.0775, 62.7933) (23.0803, 62.8999) (23.0826, 63.0066) (23.0843, 63.1134) (23.0855, 63.2203) (23.0863, 63.3273) (23.0865, 63.4344) (23.0862, 63.5417) (23.0854, 63.649) (23.0842, 63.7564) (23.0825, 63.8638) (23.0802, 63.9714) (23.0776, 64.0791) (23.0744, 64.1868) (23.0708, 64.2947) (23.0667, 64.4026) (23.0621, 64.5106) (23.0571, 64.6186) (23.0517, 64.7268) (23.0458, 64.835) (23.0394, 64.9433) (23.0326, 65.0516) (23.0254, 65.16) (23.0177, 65.2685) (23.0096, 65.3771) (23.0011, 65.4857) (22.9921, 65.5944) (22.9828, 65.7031) (22.9729, 65.8119) (22.9627, 65.9207) (22.9521, 66.0296) (22.941, 66.1386) (22.9295, 66.2476) (22.9177, 66.3567) (22.9054, 66.4658) (22.8952, 66.5531) (22.8874, 66.6186) (22.8821, 66.6623) (22.8795, 66.6842) knots 0.21931 0.21931 0.21931 0.21931 0.21931 0.21931 0.228571 0.242857 0.257143 0.271429 0.285714 0.3 0.314286 0.328571 0.342857 0.357143 0.371429 0.385714 0.4 0.414286 0.428571 0.442857 0.457143 0.471429 0.485714 0.5 0.514286 0.528571 0.542857 0.557143 0.571429 0.585714 0.6 0.614286 0.628571 0.642857 0.657143 0.671429 0.685714 0.7 0.714286 0.728571 0.742857 0.757143 0.771429 0.785714 0.8 0.814286 0.828571 0.842857 0.857143 0.871429 0.885714 0.9 0.914286 0.928571 0.942857 0.957143 0.971429 0.985714 1 1 1 1 1 1
  arc A19 (22.8795, 66.6842) -> (20.6861, 67.3969) centre (0, 0) ccw
  spline S38 degree 5 poles (20.6861, 67.3969) (20.6711, 67.3807) (20.6411, 67.3485) (20.5963, 67.3001) (20.5368, 67.2354) (20.4627, 67.1543) (20.389, 67.0731) (20.3156, 66.9916) (20.2426, 66.91) (20.17, 66.8281) (20.0978, 66.7461) (20.0259, 66.6638) (19.9544, 66.5814) (19.8832, 66.4987) (19.8125, 66.4159) (19.7421, 66.3328) (19.6722, 66.2496) (19.6026, 66.1661) (19.5334, 66.0824) (19.4646, 65.9986) (19.3962, 65.9145) (19.3283, 65.8302) (19.2607, 65.7457) (19.1935, 65.661) (19.1268, 65.5761) (19.0605, 65.491) (18.9946, 65.4057) (18.9291, 65.3202) (18.8641, 65.2345) (18.7995, 65.1485) (18.7354, 65.0624) (18.6717, 64.976) (18.6085, 64.8894) (18.5457, 64.8027) (18.4834, 64.7157) (18.4215, 64.6284) (18.3602, 64.541) (18.2993, 64.4534) (18.2389, 64.3655) (18.179, 64.2774) (18.1196, 64.1891) (18.0608, 64.1006) (18.0024, 64.0118) (17.9446, 63.9228) (17.8872, 63.8336) (17.8305, 63.7442) (17.7743, 63.6545) (17.7187, 63.5646) (17.6636, 63.4745) (17.6092, 63.3841) (17.5553, 63.2935) (17.502, 63.2026) (17.4494, 63.1115) (17.3973, 63.0202) (17.346, 62.9285) (17.2989, 62.8431) (17.2624, 62.7759) (17.2361, 62.727) (17.2199, 62.6966) (17.2135, 62.6846) knots -1 -1 -1 -1 -1 -1 -0.985714 -0.971429 -0.957143 -0.942857 -0.928571 -0.914286 -0.9 -0.885714 -0.871429 -0.857143 -0.842857 -0.828571 -0.814286 -0.8 -0.785714 -0.771429 -0.757143 -0.742857 -0.728571 -0.714286 -0.7 -0.685714 -0.671429 -0.657143 -0.642857 -0.628571 -0.614286 -0.6 -0.585714 -0.571429 -0.557143 -0.542857 -0.528571 -0.514286 -0.5 -0.485714 -0.471429 -0.457143 -0.442857 -0.428571 -0.414286 -0.4 -0.385714 -0.371429 -0.357143 -0.342857 -0.328571 -0.314286 -0.3 -0.285714 -0.271429 -0.257143 -0.242857 -0.228571 -0.21931 -0.21931 -0.21931 -0.21931 -0.21931 -0.21931
  spline S39 degree 3 poles (15.5241, 61.9332) (15.7135, 61.8857) (15.9105, 61.8757) (16.2971, 61.9317) (16.4831, 61.9972) (16.7697, 62.1664) (16.878, 62.2522) (17.0681, 62.4511) (17.149, 62.5631) (17.2135, 62.6846) knots 0 0 0 0 0.058597 0.058597 0.117193 0.117193 0.158456 0.158456 0.199718 0.199718 0.199718 0.199718
  arc A20 (15.5241, 61.9332) -> (15.3689, 61.9719) centre (0, 0) ccw
  spline S40 degree 3 poles (14.23, 63.4285) (14.2299, 63.2331) (14.268, 63.0397) (14.4161, 62.6782) (14.5248, 62.5137) (14.7585, 62.2767) (14.8681, 62.1925) (15.1071, 62.0563) (15.2354, 62.005) (15.3689, 61.9719) knots 0 0 0 0 0.058597 0.058597 0.117193 0.117193 0.158456 0.158456 0.199718 0.199718 0.199718 0.199718